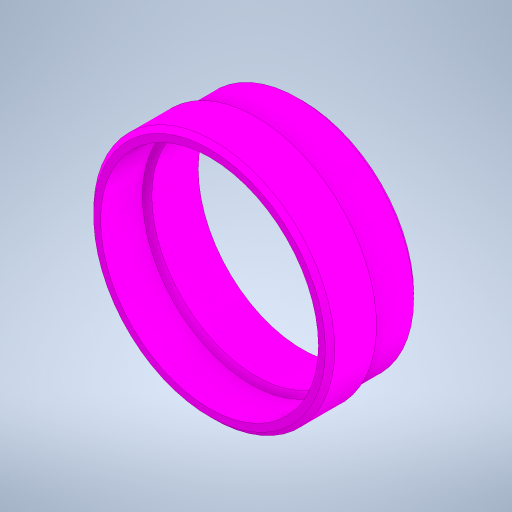
# Autodesk Inventor part: Camera Mount Adapter
Saved by Autodesk Inventor 2023.1 (Build 271208000, 208)
## iProperties
Created: 2022-11-27
Part Number: Camera Mount Adapter
Material: Generic
Document SubType Name: Modeling
Designer: xSibe
Density: 1 g/cm^3
Appearance: Plastic Magenta
Author: xSibe
Autodesk Inventor part; units mm, degrees
ref_plane "YZ Plane" through (0, 0, 0) normal (1, 0, 0) x (0, 1, 0)
ref_plane "XZ Plane" through (0, 0, 0) normal (0, 1, 0) x (-1, 0, 0)
ref_plane "XY Plane" through (0, 0, 0) normal (0, 0, 1) x (1, 0, 0)
sketch "Sketch1" plane through (0, 0, 0) normal (0, 0, 1) x (1, 0, 0)
  circle A0 centre (0, 0) radius 12.4625
  circle A1 centre (0, 0) radius 12.9625
  circle A2 centre (0, 0) radius 11.7125
  circle A3 centre (0, 0) radius 11.2125
  dimension "d0" = 24.925
  dimension "d1" = 25.925
  dimension "d2" = 1.25
  dimension "d3" = 1.25
  constraints: 4 centre point, 2 coincident
  measures "d0" diameter of A0
  measures "d1" diameter of A1
  measures "d2" radial gap between concentric circles of A1 A2
  measures "d3" radial gap between concentric circles of A0 A3
extrude "Extrusion1" add sketch "Sketch1" along normal blind 5 contours A0 | A1
extrude "Extrusion2" add sketch "Sketch1" against normal blind 5 contours A0 | A2
chamfer "Chamfer1" distance 0.5 angle 45 1 edges at (-11.7125, 0, 0)
chamfer "Chamfer2" distance 0.5 angle 45 2 edges at (-12.4625, 0, -5) (-12.9625, 0, 5)
body "Solid1"
